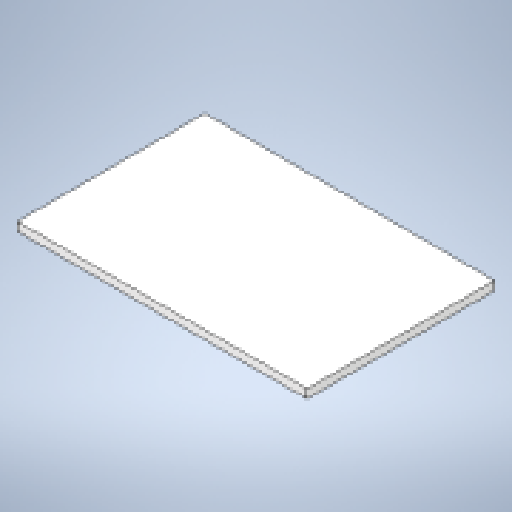
# Autodesk Inventor part: Ramp
Saved by Autodesk Inventor 2023.2 (Build 272271000, 271)
## iProperties
Created: 2024-01-21
Part Number: Ramp
Material: UHMW, White
Document SubType Name: Modeling
Designer: Nathan Cai
Mass: 22.504 g
Surface Area: 162.096 cm^2
Volume: 23.9405 cm^3
Density: 0.94 g/cm^3
Appearance: Smooth - White
Author: Nathan Cai
Autodesk Inventor part; units mm, degrees
ref_plane "YZ Plane" through (0, 0, 0) normal (1, 0, 0) x (0, 1, 0)
ref_plane "XZ Plane" through (0, 0, 0) normal (0, 1, 0) x (-1, 0, 0)
ref_plane "XY Plane" through (0, 0, 0) normal (0, 0, 1) x (1, 0, 0)
sketch "Sketch1" plane through (0, 0, 0) normal (0, 1, 0) x (-1, 0, 0)
  line L0 (-53.975, 34.925) -> (53.975, 34.925)
  line L1 (53.975, 34.925) -> (53.975, -34.925)
  line L2 (53.975, -34.925) -> (-53.975, -34.925)
  line L3 (-53.975, -34.925) -> (-53.975, 34.925)
  line L4 (-53.975, 34.925) -> (53.975, -34.925) construction
  line L5 (53.975, 34.925) -> (-53.975, -34.925) construction
  point P0 (0, 0)
  dimension "d0" = 107.95
  dimension "d1" = 69.85
  constraints: 12 end point, 2 midpoint, 2 parallel, 1 horizontal, 1 perpendicular
  measures "d0" distance of L1.end L2.end
  measures "d1" distance of L0.end L1.end
extrude "Extrusion1" add sketch "Sketch1" along normal blind 3.175
body "Solid1"
